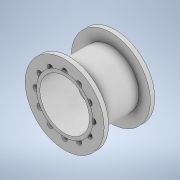
# Autodesk Inventor part: Spool
Saved by Autodesk Inventor 2020.2 (Build 242310000, 310)
## iProperties
Created: 2020-03-11
Part Number: Spool
Material: Generic
Document SubType Name: Modeling
Designer: elmar
Density: 1 g/cm^3
Appearance: Default
Author: elmar
Autodesk Inventor part; units mm, degrees
ref_plane "YZ Plane" through (0, 0, 0) normal (1, 0, 0) x (0, 1, 0)
ref_plane "XZ Plane" through (0, 0, 0) normal (0, 1, 0) x (-1, 0, 0)
ref_plane "XY Plane" through (0, 0, 0) normal (0, 0, 1) x (1, 0, 0)
sketch "Sketch1" plane through (0, 0, 0) normal (0, 0, 1) x (1, 0, 0)
  circle A0 centre (0, 0) radius 10
  dimension "d0" = 20
  constraints: 1 centre point, 1 coincident
  measures "d0" diameter of A0
extrude "Extrusion1" add sketch "Sketch1" along normal mid plane 18
sketch "Sketch2" plane through (0, 0, -9) normal (0, 0, -1) x (-1, 0, 0)
  point P0 (0, 0)
hole "Hole1" at (0, 0, -9) direction (0, 0, 1) diameter 3.2 end through all clearance for "Flat Head Machine Screw" size "M3" standard "Ansi Metric M Profile"
sketch "Sketch3" plane through (0, 0, 9) normal (0, 0, 1) x (1, 0, 0)
  circle A0 centre (0, 0) radius 14
  circle A1 centre (0, 0) radius 10 projected
  dimension "d10" = 28
  constraints: 1 centre point, 1 coincident
  measures "d10" diameter of A0
extrude "Extrusion2" add sketch "Sketch3" against normal blind 1.6
mirror "Mirror1" about plane through (0, 0, 0) normal (0, 0, 1) of "Extrusion2"
sketch "Sketch4" plane through (0, 0, 9) normal (0, 0, 1) x (1, 0, 0)
  circle A0 centre (0, 0) radius 10 projected
  circle A1 centre (0, 0) radius 10 projected
  circle A2 centre (0, 0) radius 1.6 projected
  circle A3 centre (0, 0) radius 8.8
  circle A4 centre (0, 0) radius 3.6
  dimension "d13" = 1.2
  dimension "d14" = 2
  constraints: 2 centre point
  measures "d13" radial gap between concentric circles of A3 A0
  measures "d14" radial gap between concentric circles of A2 A4
extrude "Extrusion3" cut sketch "Sketch4" against normal up to surface (16.4 mm away) contours A3
sketch "Sketch5" plane through (0, 0, 9) normal (0, 0, 1) x (1, 0, 0)
  circle A0 centre (0, 0) radius 3.6 projected
extrude "Extrusion4" cut sketch "Sketch5" against normal blind 8.4
sketch "Sketch6" plane through (0, 0, -7.4) normal (0, 0, 1) x (1, 0, 0)
  circle A0 centre (0, 0) radius 14 projected
  circle A1 centre (0, 0) radius 10 projected
  circle A2 centre (0, 0) radius 13.2
  dimension "d19" = 0.8
  constraints: 1 centre point
  measures "d19" radial gap between concentric circles of A2 A0
extrude "PrintingSupport" [suppressed]
sketch "Sketch7" plane through (0, 0, -9) normal (0, 0, -1) x (-1, 0, 0)
  circle A0 centre (0, 0) radius 10 projected
surface extrude "ExtrusionSrf1" sketch "Sketch7" against normal through all shown no curves A0
split body "Split1" result two bodies by surface "ExtrusionSrf1" first body at (12.4342, -1.9145, -7.9) (12.4342, -1.9145, 7.9)
split body "Split2" result two bodies by plane through (0, 0, 0) normal (0, 0, 1) bodies 2 first body at (12.4342, -1.9145, 7.9)
combine bodies "Combine1" operation type add bodies to combine 3 5
sketch "Sketch8" plane through (0, 0, 9) normal (0, 0, 1) x (1, 0, 0)
  line L0 (-1, 9.9499) -> (-1, 10.1999)
  line L1 (1, 9.9499) -> (1, 10.1999)
  arc A0 (1, 10.1999) -> (-1, 10.1999) centre (0, 10.1999) ccw
  line L2 (0, -19.6) -> (0, 19.6) projected
  circle A1 centre (0, 0) radius 10 projected
  dimension "d24" = 1
  dimension "d25" = 0.25
  constraints: 4 end point, 4 point on circle, 2 tangent, 2 vertical, 1 centre point, 1 point on line
  measures "d24" radius of A0
  measures "d25" distance of L0.start L0.end
extrude "Extrusion6" cut sketch "Sketch8" against normal through all contours L0 A0 L2 A1 | L2 A0 L1 A1 bodies 4
pattern_circular "Circular Pattern1" count 12 over 360 about axis through (0, 0, -10) along (0, 0, 1) of "Extrusion6" bodies 4
body "Srf1"
